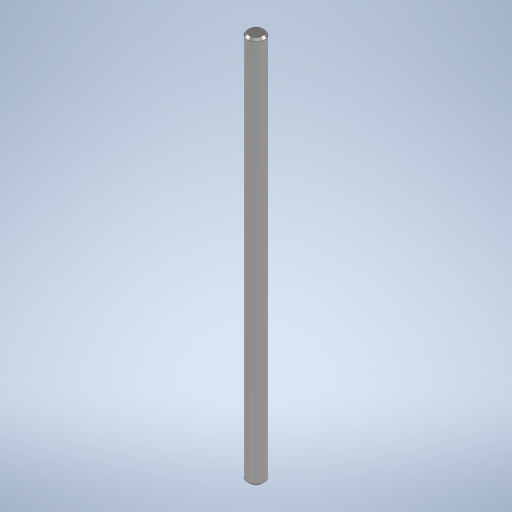
# Autodesk Inventor part: Val340
Saved by Autodesk Inventor 2024 (Build 280153000, 153)
## iProperties
Created: 2023-08-21
Part Number: Val340
Material: Steel, Cast
Document SubType Name: Modeling
Designer: KirikDK
Mass: 566.754 g
Surface Area: 183.695 cm^2
Volume: 72.198 cm^3
Density: 7.85 g/cm^3
Appearance: Semi-Polished
Author: KirikDK
Autodesk Inventor part; units mm, degrees
ref_plane "YZ Plane" through (0, 0, 0) normal (1, 0, 0) x (0, 1, 0)
ref_plane "XZ Plane" through (0, 0, 0) normal (0, 1, 0) x (-1, 0, 0)
ref_plane "XY Plane" through (0, 0, 0) normal (0, 0, 1) x (1, 0, 0)
sketch "Sketch1" plane through (0, 0, 0) normal (0, 1, 0) x (-1, 0, 0)
  circle A0 centre (0, 0) radius 8
  dimension "d0" = 16
  constraints: 1 centre point, 1 coincident
  measures "d0" diameter of A0
extrude "Extrusion1" add sketch "Sketch1" along normal blind 360
chamfer "Chamfer1" distance 2 angle 45 2 edges at (8, 360, 0) (8, 0, 0)
body "Solid1"
